Autodesk Inventor part; units mm, degrees
(part 2 of 2)
sketch "Sketch8" plane through (0, 0, 9) normal (0, 0, -1) x (-1, 0, 0)
  circle A0 centre (-8.9909, 76.1845) radius 2.5 projected
  circle A1 centre (-46.3909, 76.1845) radius 2.5 projected
  circle A2 centre (-27.6909, 76.1845) radius 2.5 projected
  arc A3 (-14.3665, 90.3268) -> (-12.2661, 92.4931) centre (-15.59, 93.6145) ccw projected
  arc A4 (-14.955, 86.1395) -> (-14.3665, 90.3268) centre (-14.955, 88.2745) ccw projected
  line L0 (-17.86, 86.1395) -> (-14.955, 86.1395) projected
  line L1 (-17.86, 86.6395) -> (-17.86, 86.1395) projected
  line L2 (-14.955, 86.6395) -> (-17.86, 86.6395) projected
  arc A5 (-14.955, 86.6395) -> (-14.955, 89.9095) centre (-14.955, 88.2745) ccw projected
  line L3 (-16.225, 89.9095) -> (-14.955, 89.9095) projected
  arc A6 (-16.7766, 90.8591) -> (-16.225, 89.9095) centre (-16.225, 90.5445) ccw projected
  arc A7 (-16.7766, 90.8591) -> (-12.6611, 92.9653) centre (-15.59, 93.6145) ccw projected
  arc A8 (-12.6611, 92.9653) -> (-11.1978, 95.4171) centre (-12.6138, 94.5996) ccw projected
  line L4 (-11.8328, 96.5169) -> (-11.1978, 95.4171) projected
  arc A9 (-10.733, 97.1519) -> (-11.8328, 96.5169) centre (-11.2829, 96.8344) ccw projected
  line L5 (-9.2805, 94.6361) -> (-10.733, 97.1519) projected
  line L6 (-9.7135, 94.3861) -> (-9.2805, 94.6361) projected
  line L7 (-11.157, 93.0388) -> (-9.7135, 94.3861) projected
  arc A10 (-12.2661, 92.4931) -> (-11.157, 93.0388) centre (-12.6138, 94.5996) ccw projected
  arc A11 (-19.049, 94.1988) -> (-18.2231, 91.2966) centre (-15.59, 93.6145) ccw projected
  arc A12 (-22.3811, 96.8021) -> (-19.049, 94.1988) centre (-20.5321, 95.7346) ccw projected
  line L8 (-20.9286, 99.3179) -> (-22.3811, 96.8021) projected
  line L9 (-20.4955, 99.0679) -> (-20.9286, 99.3179) projected
  line L10 (-21.948, 96.5521) -> (-20.4955, 99.0679) projected
  arc A13 (-21.948, 96.5521) -> (-19.1161, 94.9171) centre (-20.5321, 95.7346) ccw projected
  line L11 (-18.4811, 96.0169) -> (-19.1161, 94.9171) projected
  arc A14 (-17.3829, 96.0198) -> (-18.4811, 96.0169) centre (-17.9312, 95.6994) ccw projected
  arc A15 (-17.3829, 96.0198) -> (-17.6167, 91.4026) centre (-15.59, 93.6145) ccw projected
  arc A16 (-17.6167, 91.4026) -> (-16.225, 88.9095) centre (-16.225, 90.5445) ccw projected
  line L12 (-14.955, 88.9095) -> (-16.225, 88.9095) projected
  arc A17 (-14.955, 87.6395) -> (-14.955, 88.9095) centre (-14.955, 88.2745) ccw projected
  line L13 (-17.86, 87.6395) -> (-14.955, 87.6395) projected
  line L14 (-17.86, 88.1395) -> (-17.86, 87.6395) projected
  line L15 (-18.3051, 90.0633) -> (-17.86, 88.1395) projected
  arc A18 (-18.2231, 91.2966) -> (-18.3051, 90.0633) centre (-16.225, 90.5445) ccw projected
  arc A19 (-13.3545, 96.3179) -> (-16.2808, 97.0538) centre (-15.59, 93.6145) ccw projected
  arc A20 (-9.4339, 97.9019) -> (-13.3545, 96.3179) centre (-11.2829, 96.8344) ccw projected
  line L16 (-7.9814, 95.3861) -> (-9.4339, 97.9019) projected
  line L17 (-8.4145, 95.1361) -> (-7.9814, 95.3861) projected
  line L18 (-9.867, 97.6519) -> (-8.4145, 95.1361) projected
  arc A21 (-9.867, 97.6519) -> (-12.6989, 96.0169) centre (-11.2829, 96.8344) ccw projected
  line L19 (-12.0639, 94.9171) -> (-12.6989, 96.0169) projected
  arc A22 (-12.6105, 93.9646) -> (-12.0639, 94.9171) centre (-12.6138, 94.5996) ccw projected
  arc A23 (-12.6105, 93.9646) -> (-16.4922, 96.4756) centre (-15.59, 93.6145) ccw projected
  arc A24 (-16.4922, 96.4756) -> (-19.3472, 96.5169) centre (-17.9312, 95.6994) ccw projected
  line L20 (-19.9822, 95.4171) -> (-19.3472, 96.5169) projected
  arc A25 (-21.082, 96.0521) -> (-19.9822, 95.4171) centre (-20.5321, 95.7346) ccw projected
  line L21 (-19.6295, 98.5679) -> (-21.082, 96.0521) projected
  line L22 (-19.1965, 98.3179) -> (-19.6295, 98.5679) projected
  line L23 (-17.3079, 97.7414) -> (-19.1965, 98.3179) projected
  arc A26 (-16.2808, 97.0538) -> (-17.3079, 97.7414) centre (-17.9312, 95.6994) ccw projected
  arc A27 (-33.0665, 90.3268) -> (-30.9661, 92.4931) centre (-34.29, 93.6145) ccw projected
  arc A28 (-33.655, 86.1395) -> (-33.0665, 90.3268) centre (-33.655, 88.2745) ccw projected
  line L24 (-36.56, 86.1395) -> (-33.655, 86.1395) projected
  line L25 (-36.56, 86.6395) -> (-36.56, 86.1395) projected
  line L26 (-33.655, 86.6395) -> (-36.56, 86.6395) projected
  arc A29 (-33.655, 86.6395) -> (-33.655, 89.9095) centre (-33.655, 88.2745) ccw projected
  line L27 (-34.925, 89.9095) -> (-33.655, 89.9095) projected
  arc A30 (-35.4766, 90.8591) -> (-34.925, 89.9095) centre (-34.925, 90.5445) ccw projected
  arc A31 (-35.4766, 90.8591) -> (-31.3611, 92.9653) centre (-34.29, 93.6145) ccw projected
  arc A32 (-31.3611, 92.9653) -> (-29.8978, 95.4171) centre (-31.3138, 94.5996) ccw projected
  line L28 (-30.5328, 96.5169) -> (-29.8978, 95.4171) projected
  arc A33 (-29.433, 97.1519) -> (-30.5328, 96.5169) centre (-29.9829, 96.8344) ccw projected
  line L29 (-27.9805, 94.6361) -> (-29.433, 97.1519) projected
  line L30 (-28.4135, 94.3861) -> (-27.9805, 94.6361) projected
  line L31 (-29.857, 93.0388) -> (-28.4135, 94.3861) projected
  arc A34 (-30.9661, 92.4931) -> (-29.857, 93.0388) centre (-31.3138, 94.5996) ccw projected
  arc A35 (-37.749, 94.1988) -> (-36.9231, 91.2966) centre (-34.29, 93.6145) ccw projected
  arc A36 (-41.0811, 96.8021) -> (-37.749, 94.1988) centre (-39.2321, 95.7346) ccw projected
  line L32 (-39.6286, 99.3179) -> (-41.0811, 96.8021) projected
  line L33 (-39.1955, 99.0679) -> (-39.6286, 99.3179) projected
  line L34 (-40.648, 96.5521) -> (-39.1955, 99.0679) projected
  arc A37 (-40.648, 96.5521) -> (-37.8161, 94.9171) centre (-39.2321, 95.7346) ccw projected
  line L35 (-37.1811, 96.0169) -> (-37.8161, 94.9171) projected
  arc A38 (-36.0829, 96.0198) -> (-37.1811, 96.0169) centre (-36.6312, 95.6994) ccw projected
  arc A39 (-36.0829, 96.0198) -> (-36.3167, 91.4026) centre (-34.29, 93.6145) ccw projected
  arc A40 (-36.3167, 91.4026) -> (-34.925, 88.9095) centre (-34.925, 90.5445) ccw projected
  line L36 (-33.655, 88.9095) -> (-34.925, 88.9095) projected
  arc A41 (-33.655, 87.6395) -> (-33.655, 88.9095) centre (-33.655, 88.2745) ccw projected
  line L37 (-36.56, 87.6395) -> (-33.655, 87.6395) projected
  line L38 (-36.56, 88.1395) -> (-36.56, 87.6395) projected
  line L39 (-37.0051, 90.0633) -> (-36.56, 88.1395) projected
  arc A42 (-36.9231, 91.2966) -> (-37.0051, 90.0633) centre (-34.925, 90.5445) ccw projected
  arc A43 (-32.0545, 96.3179) -> (-34.9808, 97.0538) centre (-34.29, 93.6145) ccw projected
  arc A44 (-28.1339, 97.9019) -> (-32.0545, 96.3179) centre (-29.9829, 96.8344) ccw projected
  line L40 (-26.6814, 95.3861) -> (-28.1339, 97.9019) projected
  line L41 (-27.1145, 95.1361) -> (-26.6814, 95.3861) projected
  line L42 (-28.567, 97.6519) -> (-27.1145, 95.1361) projected
  arc A45 (-28.567, 97.6519) -> (-31.3989, 96.0169) centre (-29.9829, 96.8344) ccw projected
  line L43 (-30.7639, 94.9171) -> (-31.3989, 96.0169) projected
  arc A46 (-31.3105, 93.9646) -> (-30.7639, 94.9171) centre (-31.3138, 94.5996) ccw projected
  arc A47 (-31.3105, 93.9646) -> (-35.1922, 96.4756) centre (-34.29, 93.6145) ccw projected
  arc A48 (-35.1922, 96.4756) -> (-38.0472, 96.5169) centre (-36.6312, 95.6994) ccw projected
  line L44 (-38.6822, 95.4171) -> (-38.0472, 96.5169) projected
  arc A49 (-39.782, 96.0521) -> (-38.6822, 95.4171) centre (-39.2321, 95.7346) ccw projected
  line L45 (-38.3295, 98.5679) -> (-39.782, 96.0521) projected
  line L46 (-37.8965, 98.3179) -> (-38.3295, 98.5679) projected
  line L47 (-36.0079, 97.7414) -> (-37.8965, 98.3179) projected
  arc A50 (-34.9808, 97.0538) -> (-36.0079, 97.7414) centre (-36.6312, 95.6994) ccw projected
  arc A51 (-51.7665, 90.3268) -> (-49.6661, 92.4931) centre (-52.99, 93.6145) ccw projected
  arc A52 (-52.355, 86.1395) -> (-51.7665, 90.3268) centre (-52.355, 88.2745) ccw projected
  line L48 (-55.26, 86.1395) -> (-52.355, 86.1395) projected
  line L49 (-55.26, 86.6395) -> (-55.26, 86.1395) projected
  line L50 (-52.355, 86.6395) -> (-55.26, 86.6395) projected
  arc A53 (-52.355, 86.6395) -> (-52.355, 89.9095) centre (-52.355, 88.2745) ccw projected
  line L51 (-53.625, 89.9095) -> (-52.355, 89.9095) projected
  arc A54 (-54.1766, 90.8591) -> (-53.625, 89.9095) centre (-53.625, 90.5445) ccw projected
  arc A55 (-54.1766, 90.8591) -> (-50.0611, 92.9653) centre (-52.99, 93.6145) ccw projected
  arc A56 (-50.0611, 92.9653) -> (-48.5978, 95.4171) centre (-50.0138, 94.5996) ccw projected
  line L52 (-49.2328, 96.5169) -> (-48.5978, 95.4171) projected
  arc A57 (-48.133, 97.1519) -> (-49.2328, 96.5169) centre (-48.6829, 96.8344) ccw projected
  line L53 (-46.6805, 94.6361) -> (-48.133, 97.1519) projected
  line L54 (-47.1135, 94.3861) -> (-46.6805, 94.6361) projected
  line L55 (-48.557, 93.0388) -> (-47.1135, 94.3861) projected
  arc A58 (-49.6661, 92.4931) -> (-48.557, 93.0388) centre (-50.0138, 94.5996) ccw projected
  arc A59 (-56.449, 94.1988) -> (-55.6231, 91.2966) centre (-52.99, 93.6145) ccw projected
  arc A60 (-59.7811, 96.8021) -> (-56.449, 94.1988) centre (-57.9321, 95.7346) ccw projected
  line L56 (-58.3286, 99.3179) -> (-59.7811, 96.8021) projected
  line L57 (-57.8955, 99.0679) -> (-58.3286, 99.3179) projected
  line L58 (-59.348, 96.5521) -> (-57.8955, 99.0679) projected
  arc A61 (-59.348, 96.5521) -> (-56.5161, 94.9171) centre (-57.9321, 95.7346) ccw projected
  line L59 (-55.8811, 96.0169) -> (-56.5161, 94.9171) projected
  arc A62 (-54.7829, 96.0198) -> (-55.8811, 96.0169) centre (-55.3312, 95.6994) ccw projected
  arc A63 (-54.7829, 96.0198) -> (-55.0167, 91.4026) centre (-52.99, 93.6145) ccw projected
  arc A64 (-55.0167, 91.4026) -> (-53.625, 88.9095) centre (-53.625, 90.5445) ccw projected
  line L60 (-52.355, 88.9095) -> (-53.625, 88.9095) projected
  arc A65 (-52.355, 87.6395) -> (-52.355, 88.9095) centre (-52.355, 88.2745) ccw projected
  line L61 (-55.26, 87.6395) -> (-52.355, 87.6395) projected
  line L62 (-55.26, 88.1395) -> (-55.26, 87.6395) projected
  line L63 (-55.7051, 90.0633) -> (-55.26, 88.1395) projected
  arc A66 (-55.6231, 91.2966) -> (-55.7051, 90.0633) centre (-53.625, 90.5445) ccw projected
  arc A67 (-50.7545, 96.3179) -> (-53.6808, 97.0538) centre (-52.99, 93.6145) ccw projected
  arc A68 (-46.8339, 97.9019) -> (-50.7545, 96.3179) centre (-48.6829, 96.8344) ccw projected
  line L64 (-45.3814, 95.3861) -> (-46.8339, 97.9019) projected
  line L65 (-45.8145, 95.1361) -> (-45.3814, 95.3861) projected
  line L66 (-47.267, 97.6519) -> (-45.8145, 95.1361) projected
  arc A69 (-47.267, 97.6519) -> (-50.0989, 96.0169) centre (-48.6829, 96.8344) ccw projected
  line L67 (-49.4639, 94.9171) -> (-50.0989, 96.0169) projected
  arc A70 (-50.0105, 93.9646) -> (-49.4639, 94.9171) centre (-50.0138, 94.5996) ccw projected
  arc A71 (-50.0105, 93.9646) -> (-53.8922, 96.4756) centre (-52.99, 93.6145) ccw projected
  arc A72 (-53.8922, 96.4756) -> (-56.7472, 96.5169) centre (-55.3312, 95.6994) ccw projected
  line L68 (-57.3822, 95.4171) -> (-56.7472, 96.5169) projected
  arc A73 (-58.482, 96.0521) -> (-57.3822, 95.4171) centre (-57.9321, 95.7346) ccw projected
  line L69 (-57.0295, 98.5679) -> (-58.482, 96.0521) projected
  line L70 (-56.5965, 98.3179) -> (-57.0295, 98.5679) projected
  line L71 (-54.7079, 97.7414) -> (-56.5965, 98.3179) projected
  arc A74 (-53.6808, 97.0538) -> (-54.7079, 97.7414) centre (-55.3312, 95.6994) ccw projected
  arc A75 (-14.3665, 76.7068) -> (-12.2661, 78.8731) centre (-15.59, 79.9945) ccw projected
  arc A76 (-14.955, 72.5195) -> (-14.3665, 76.7068) centre (-14.955, 74.6545) ccw projected
  line L72 (-17.86, 72.5195) -> (-14.955, 72.5195) projected
  line L73 (-17.86, 73.0195) -> (-17.86, 72.5195) projected
  line L74 (-14.955, 73.0195) -> (-17.86, 73.0195) projected
  arc A77 (-14.955, 73.0195) -> (-14.955, 76.2895) centre (-14.955, 74.6545) ccw projected
  line L75 (-16.225, 76.2895) -> (-14.955, 76.2895) projected
  arc A78 (-16.7766, 77.2391) -> (-16.225, 76.2895) centre (-16.225, 76.9245) ccw projected
  arc A79 (-16.7766, 77.2391) -> (-12.6611, 79.3453) centre (-15.59, 79.9945) ccw projected
  arc A80 (-12.6611, 79.3453) -> (-11.1978, 81.7971) centre (-12.6138, 80.9796) ccw projected
  line L76 (-11.8328, 82.8969) -> (-11.1978, 81.7971) projected
  arc A81 (-10.733, 83.5319) -> (-11.8328, 82.8969) centre (-11.2829, 83.2144) ccw projected
  line L77 (-9.2805, 81.0161) -> (-10.733, 83.5319) projected
  line L78 (-9.7135, 80.7661) -> (-9.2805, 81.0161) projected
  line L79 (-11.157, 79.4188) -> (-9.7135, 80.7661) projected
  arc A82 (-12.2661, 78.8731) -> (-11.157, 79.4188) centre (-12.6138, 80.9796) ccw projected
  arc A83 (-19.049, 80.5788) -> (-18.2231, 77.6766) centre (-15.59, 79.9945) ccw projected
  arc A84 (-22.3811, 83.1821) -> (-19.049, 80.5788) centre (-20.5321, 82.1146) ccw projected
  line L80 (-20.9286, 85.6979) -> (-22.3811, 83.1821) projected
  line L81 (-20.4955, 85.4479) -> (-20.9286, 85.6979) projected
  line L82 (-21.948, 82.9321) -> (-20.4955, 85.4479) projected
  arc A85 (-21.948, 82.9321) -> (-19.1161, 81.2971) centre (-20.5321, 82.1146) ccw projected
  line L83 (-18.4811, 82.3969) -> (-19.1161, 81.2971) projected
  arc A86 (-17.3829, 82.3998) -> (-18.4811, 82.3969) centre (-17.9312, 82.0794) ccw projected
  arc A87 (-17.3829, 82.3998) -> (-17.6167, 77.7826) centre (-15.59, 79.9945) ccw projected
  arc A88 (-17.6167, 77.7826) -> (-16.225, 75.2895) centre (-16.225, 76.9245) ccw projected
  line L84 (-14.955, 75.2895) -> (-16.225, 75.2895) projected
  arc A89 (-14.955, 74.0195) -> (-14.955, 75.2895) centre (-14.955, 74.6545) ccw projected
  line L85 (-17.86, 74.0195) -> (-14.955, 74.0195) projected
  line L86 (-17.86, 74.5195) -> (-17.86, 74.0195) projected
  line L87 (-18.3051, 76.4433) -> (-17.86, 74.5195) projected
  arc A90 (-18.2231, 77.6766) -> (-18.3051, 76.4433) centre (-16.225, 76.9245) ccw projected
  arc A91 (-13.3545, 82.6979) -> (-16.2808, 83.4338) centre (-15.59, 79.9945) ccw projected
  arc A92 (-9.4339, 84.2819) -> (-13.3545, 82.6979) centre (-11.2829, 83.2144) ccw projected
  line L88 (-7.9814, 81.7661) -> (-9.4339, 84.2819) projected
  line L89 (-8.4145, 81.5161) -> (-7.9814, 81.7661) projected
  line L90 (-9.867, 84.0319) -> (-8.4145, 81.5161) projected
  arc A93 (-9.867, 84.0319) -> (-12.6989, 82.3969) centre (-11.2829, 83.2144) ccw projected
  line L91 (-12.0639, 81.2971) -> (-12.6989, 82.3969) projected
  arc A94 (-12.6105, 80.3446) -> (-12.0639, 81.2971) centre (-12.6138, 80.9796) ccw projected
  arc A95 (-12.6105, 80.3446) -> (-16.4922, 82.8556) centre (-15.59, 79.9945) ccw projected
  arc A96 (-16.4922, 82.8556) -> (-19.3472, 82.8969) centre (-17.9312, 82.0794) ccw projected
  line L92 (-19.9822, 81.7971) -> (-19.3472, 82.8969) projected
  arc A97 (-21.082, 82.4321) -> (-19.9822, 81.7971) centre (-20.5321, 82.1146) ccw projected
  line L93 (-19.6295, 84.9479) -> (-21.082, 82.4321) projected
  line L94 (-19.1965, 84.6979) -> (-19.6295, 84.9479) projected
  line L95 (-17.3079, 84.1214) -> (-19.1965, 84.6979) projected
  arc A98 (-16.2808, 83.4338) -> (-17.3079, 84.1214) centre (-17.9312, 82.0794) ccw projected
  arc A99 (-33.0665, 76.7068) -> (-30.9661, 78.8731) centre (-34.29, 79.9945) ccw projected
  arc A100 (-33.655, 72.5195) -> (-33.0665, 76.7068) centre (-33.655, 74.6545) ccw projected
  line L96 (-36.56, 72.5195) -> (-33.655, 72.5195) projected
  line L97 (-36.56, 73.0195) -> (-36.56, 72.5195) projected
  line L98 (-33.655, 73.0195) -> (-36.56, 73.0195) projected
  arc A101 (-33.655, 73.0195) -> (-33.655, 76.2895) centre (-33.655, 74.6545) ccw projected
  line L99 (-34.925, 76.2895) -> (-33.655, 76.2895) projected
  arc A102 (-35.4766, 77.2391) -> (-34.925, 76.2895) centre (-34.925, 76.9245) ccw projected
  arc A103 (-35.4766, 77.2391) -> (-31.3611, 79.3453) centre (-34.29, 79.9945) ccw projected
  arc A104 (-31.3611, 79.3453) -> (-29.8978, 81.7971) centre (-31.3138, 80.9796) ccw projected
  line L100 (-30.5328, 82.8969) -> (-29.8978, 81.7971) projected
  arc A105 (-29.433, 83.5319) -> (-30.5328, 82.8969) centre (-29.9829, 83.2144) ccw projected
  line L101 (-27.9805, 81.0161) -> (-29.433, 83.5319) projected
  line L102 (-28.4135, 80.7661) -> (-27.9805, 81.0161) projected
  line L103 (-29.857, 79.4188) -> (-28.4135, 80.7661) projected
  arc A106 (-30.9661, 78.8731) -> (-29.857, 79.4188) centre (-31.3138, 80.9796) ccw projected
  arc A107 (-37.749, 80.5788) -> (-36.9231, 77.6766) centre (-34.29, 79.9945) ccw projected
  arc A108 (-41.0811, 83.1821) -> (-37.749, 80.5788) centre (-39.2321, 82.1146) ccw projected
  line L104 (-39.6286, 85.6979) -> (-41.0811, 83.1821) projected
  line L105 (-39.1955, 85.4479) -> (-39.6286, 85.6979) projected
  line L106 (-40.648, 82.9321) -> (-39.1955, 85.4479) projected
  arc A109 (-40.648, 82.9321) -> (-37.8161, 81.2971) centre (-39.2321, 82.1146) ccw projected
  line L107 (-37.1811, 82.3969) -> (-37.8161, 81.2971) projected
  arc A110 (-36.0829, 82.3998) -> (-37.1811, 82.3969) centre (-36.6312, 82.0794) ccw projected
  arc A111 (-36.0829, 82.3998) -> (-36.3167, 77.7826) centre (-34.29, 79.9945) ccw projected
  arc A112 (-36.3167, 77.7826) -> (-34.925, 75.2895) centre (-34.925, 76.9245) ccw projected
  line L108 (-33.655, 75.2895) -> (-34.925, 75.2895) projected
  arc A113 (-33.655, 74.0195) -> (-33.655, 75.2895) centre (-33.655, 74.6545) ccw projected
  line L109 (-36.56, 74.0195) -> (-33.655, 74.0195) projected
  line L110 (-36.56, 74.5195) -> (-36.56, 74.0195) projected
  line L111 (-37.0051, 76.4433) -> (-36.56, 74.5195) projected
  arc A114 (-36.9231, 77.6766) -> (-37.0051, 76.4433) centre (-34.925, 76.9245) ccw projected
  arc A115 (-32.0545, 82.6979) -> (-34.9808, 83.4338) centre (-34.29, 79.9945) ccw projected
  arc A116 (-28.1339, 84.2819) -> (-32.0545, 82.6979) centre (-29.9829, 83.2144) ccw projected
  line L112 (-26.6814, 81.7661) -> (-28.1339, 84.2819) projected
  line L113 (-27.1145, 81.5161) -> (-26.6814, 81.7661) projected
  line L114 (-28.567, 84.0319) -> (-27.1145, 81.5161) projected
  arc A117 (-28.567, 84.0319) -> (-31.3989, 82.3969) centre (-29.9829, 83.2144) ccw projected
  line L115 (-30.7639, 81.2971) -> (-31.3989, 82.3969) projected
  arc A118 (-31.3105, 80.3446) -> (-30.7639, 81.2971) centre (-31.3138, 80.9796) ccw projected
  arc A119 (-31.3105, 80.3446) -> (-35.1922, 82.8556) centre (-34.29, 79.9945) ccw projected
  arc A120 (-35.1922, 82.8556) -> (-38.0472, 82.8969) centre (-36.6312, 82.0794) ccw projected
  line L116 (-38.6822, 81.7971) -> (-38.0472, 82.8969) projected
  arc A121 (-39.782, 82.4321) -> (-38.6822, 81.7971) centre (-39.2321, 82.1146) ccw projected
  line L117 (-38.3295, 84.9479) -> (-39.782, 82.4321) projected
  line L118 (-37.8965, 84.6979) -> (-38.3295, 84.9479) projected
  line L119 (-36.0079, 84.1214) -> (-37.8965, 84.6979) projected
  arc A122 (-34.9808, 83.4338) -> (-36.0079, 84.1214) centre (-36.6312, 82.0794) ccw projected
  arc A123 (-56.449, 80.5788) -> (-55.6231, 77.6766) centre (-52.99, 79.9945) ccw projected
  arc A124 (-59.7811, 83.1821) -> (-56.449, 80.5788) centre (-57.9321, 82.1146) ccw projected
  line L120 (-58.3286, 85.6979) -> (-59.7811, 83.1821) projected
  line L121 (-57.8955, 85.4479) -> (-58.3286, 85.6979) projected
  line L122 (-59.348, 82.9321) -> (-57.8955, 85.4479) projected
  arc A125 (-59.348, 82.9321) -> (-56.5161, 81.2971) centre (-57.9321, 82.1146) ccw projected
  line L123 (-55.8811, 82.3969) -> (-56.5161, 81.2971) projected
  arc A126 (-54.7829, 82.3998) -> (-55.8811, 82.3969) centre (-55.3312, 82.0794) ccw projected
  arc A127 (-54.7829, 82.3998) -> (-55.0167, 77.7826) centre (-52.99, 79.9945) ccw projected
  arc A128 (-55.0167, 77.7826) -> (-53.625, 75.2895) centre (-53.625, 76.9245) ccw projected
  line L124 (-52.355, 75.2895) -> (-53.625, 75.2895) projected
  arc A129 (-52.355, 74.0195) -> (-52.355, 75.2895) centre (-52.355, 74.6545) ccw projected
  line L125 (-55.26, 74.0195) -> (-52.355, 74.0195) projected
  line L126 (-55.26, 74.5195) -> (-55.26, 74.0195) projected
  line L127 (-55.7051, 76.4433) -> (-55.26, 74.5195) projected
  arc A130 (-55.6231, 77.6766) -> (-55.7051, 76.4433) centre (-53.625, 76.9245) ccw projected
  arc A131 (-50.0105, 80.3446) -> (-53.8922, 82.8556) centre (-52.99, 79.9945) ccw projected
  arc A132 (-53.8922, 82.8556) -> (-56.7472, 82.8969) centre (-55.3312, 82.0794) ccw projected
  line L128 (-57.3822, 81.7971) -> (-56.7472, 82.8969) projected
  arc A133 (-58.482, 82.4321) -> (-57.3822, 81.7971) centre (-57.9321, 82.1146) ccw projected
  line L129 (-57.0295, 84.9479) -> (-58.482, 82.4321) projected
  line L130 (-56.5965, 84.6979) -> (-57.0295, 84.9479) projected
  line L131 (-54.7079, 84.1214) -> (-56.5965, 84.6979) projected
  arc A134 (-53.6808, 83.4338) -> (-54.7079, 84.1214) centre (-55.3312, 82.0794) ccw projected
  arc A135 (-50.7545, 82.6979) -> (-53.6808, 83.4338) centre (-52.99, 79.9945) ccw projected
  arc A136 (-46.8339, 84.2819) -> (-50.7545, 82.6979) centre (-48.6829, 83.2144) ccw projected
  line L132 (-45.3814, 81.7661) -> (-46.8339, 84.2819) projected
  line L133 (-45.8145, 81.5161) -> (-45.3814, 81.7661) projected
  line L134 (-47.267, 84.0319) -> (-45.8145, 81.5161) projected
  arc A137 (-47.267, 84.0319) -> (-50.0989, 82.3969) centre (-48.6829, 83.2144) ccw projected
  line L135 (-49.4639, 81.2971) -> (-50.0989, 82.3969) projected
  arc A138 (-50.0105, 80.3446) -> (-49.4639, 81.2971) centre (-50.0138, 80.9796) ccw projected
  arc A139 (-50.0611, 79.3453) -> (-48.5978, 81.7971) centre (-50.0138, 80.9796) ccw projected
  line L136 (-49.2328, 82.8969) -> (-48.5978, 81.7971) projected
  arc A140 (-48.133, 83.5319) -> (-49.2328, 82.8969) centre (-48.6829, 83.2144) ccw projected
  line L137 (-46.6805, 81.0161) -> (-48.133, 83.5319) projected
  line L138 (-47.1135, 80.7661) -> (-46.6805, 81.0161) projected
  line L139 (-48.557, 79.4188) -> (-47.1135, 80.7661) projected
  arc A141 (-49.6661, 78.8731) -> (-48.557, 79.4188) centre (-50.0138, 80.9796) ccw projected
  arc A142 (-51.7665, 76.7068) -> (-49.6661, 78.8731) centre (-52.99, 79.9945) ccw projected
  arc A143 (-52.355, 72.5195) -> (-51.7665, 76.7068) centre (-52.355, 74.6545) ccw projected
  line L140 (-55.26, 72.5195) -> (-52.355, 72.5195) projected
  line L141 (-55.26, 73.0195) -> (-55.26, 72.5195) projected
  line L142 (-52.355, 73.0195) -> (-55.26, 73.0195) projected
  arc A144 (-52.355, 73.0195) -> (-52.355, 76.2895) centre (-52.355, 74.6545) ccw projected
  line L143 (-53.625, 76.2895) -> (-52.355, 76.2895) projected
  arc A145 (-54.1766, 77.2391) -> (-53.625, 76.2895) centre (-53.625, 76.9245) ccw projected
  arc A146 (-54.1766, 77.2391) -> (-50.0611, 79.3453) centre (-52.99, 79.9945) ccw projected
  line L144 (-2, 65.8874) -> (-66.58, 65.8874) projected
  line L145 (-2, 105.95) -> (-2, 65.8874) projected
  line L146 (-66.58, 105.95) -> (-2, 105.95) projected
  line L147 (-66.58, 65.8874) -> (-66.58, 105.95) projected
  line L148 (-9.7135, 80.7661) -> (-9.2805, 81.0161) projected
  line L149 (-9.2805, 81.0161) -> (-8.4145, 81.5161)
  line L150 (-17.86, 73.0195) -> (-17.86, 72.5195) projected
  line L151 (-17.86, 74.0195) -> (-17.86, 73.0195)
  line L152 (-20.4955, 85.4479) -> (-20.9286, 85.6979) projected
  line L153 (-20.4955, 85.4479) -> (-19.6295, 84.9479)
  line L154 (-8.4145, 95.1361) -> (-7.9814, 95.3861) projected
  line L155 (-8.4145, 95.1361) -> (-9.2805, 94.6361)
  line L156 (-17.86, 86.6395) -> (-17.86, 86.1395) projected
  line L157 (-17.86, 87.6395) -> (-17.86, 86.6395)
  line L158 (-20.4955, 99.0679) -> (-19.6295, 98.5679)
  line L159 (-27.1145, 95.1361) -> (-26.6814, 95.3861) projected
  line L160 (-27.1145, 95.1361) -> (-27.9805, 94.6361)
  line L161 (-27.1145, 81.5161) -> (-27.9805, 81.0161)
  line L162 (-36.56, 73.0195) -> (-36.56, 72.5195) projected
  line L163 (-36.56, 74.0195) -> (-36.56, 73.0195)
  line L164 (-40.648, 82.9321) -> (-39.1955, 85.4479) projected
  line L165 (-38.3295, 84.9479) -> (-39.1955, 85.4479)
  line L166 (-33.655, 86.6395) -> (-36.56, 86.6395) projected
  line L167 (-36.56, 86.6395) -> (-36.56, 87.6395)
  line L168 (-40.648, 96.5521) -> (-39.1955, 99.0679) projected
  line L169 (-39.1955, 99.0679) -> (-38.3295, 98.5679)
  line L170 (-46.6805, 81.0161) -> (-45.8145, 81.5161)
  line L171 (-55.26, 73.0195) -> (-55.26, 72.5195) projected
  line L172 (-55.26, 73.0195) -> (-55.26, 74.0195)
  line L173 (-57.8955, 85.4479) -> (-57.0295, 84.9479)
  line L174 (-55.26, 87.6395) -> (-55.26, 86.6395)
  line L175 (-45.8145, 95.1361) -> (-45.3814, 95.3861) projected
  line L176 (-45.8145, 95.1361) -> (-46.6805, 94.6361)
  line L177 (-59.348, 96.5521) -> (-57.8955, 99.0679) projected
  line L178 (-57.0295, 98.5679) -> (-58.482, 96.0521) projected
  line L179 (-57.8955, 99.0679) -> (-57.0295, 98.5679)
  line L180 (-37.29, 82.9945) -> (-31.29, 82.9945)
  line L181 (-31.29, 82.9945) -> (-31.29, 76.9945)
  line L182 (-31.29, 76.9945) -> (-37.29, 76.9945)
  line L183 (-37.29, 76.9945) -> (-37.29, 82.9945)
  line L184 (-37.29, 82.9945) -> (-31.29, 76.9945) construction
  line L185 (-31.29, 82.9945) -> (-37.29, 76.9945) construction
  line L186 (-37.29, 96.6145) -> (-31.29, 96.6145)
  line L187 (-31.29, 96.6145) -> (-31.29, 90.6145)
  line L188 (-31.29, 90.6145) -> (-37.29, 90.6145)
  line L189 (-37.29, 90.6145) -> (-37.29, 96.6145)
  line L190 (-37.29, 96.6145) -> (-31.29, 90.6145) construction
  line L191 (-31.29, 96.6145) -> (-37.29, 90.6145) construction
  line L192 (-12.59, 96.6145) -> (-18.59, 96.6145)
  line L193 (-18.59, 96.6145) -> (-18.59, 90.6145)
  line L194 (-18.59, 90.6145) -> (-12.59, 90.6145)
  line L195 (-12.59, 90.6145) -> (-12.59, 96.6145)
  line L196 (-12.59, 96.6145) -> (-18.59, 90.6145) construction
  line L197 (-18.59, 96.6145) -> (-12.59, 90.6145) construction
  line L198 (-12.59, 82.9945) -> (-18.59, 82.9945)
  line L199 (-18.59, 82.9945) -> (-18.59, 76.9945)
  line L200 (-18.59, 76.9945) -> (-12.59, 76.9945)
  line L201 (-12.59, 76.9945) -> (-12.59, 82.9945)
  line L202 (-12.59, 82.9945) -> (-18.59, 76.9945) construction
  line L203 (-18.59, 82.9945) -> (-12.59, 76.9945) construction
  line L204 (-49.99, 82.9945) -> (-55.99, 82.9945)
  line L205 (-55.99, 82.9945) -> (-55.99, 76.9945)
  line L206 (-55.99, 76.9945) -> (-49.99, 76.9945)
  line L207 (-49.99, 76.9945) -> (-49.99, 82.9945)
  line L208 (-49.99, 82.9945) -> (-55.99, 76.9945) construction
  line L209 (-55.99, 82.9945) -> (-49.99, 76.9945) construction
  line L210 (-49.99, 96.6145) -> (-55.99, 96.6145)
  line L211 (-55.99, 96.6145) -> (-55.99, 90.6145)
  line L212 (-55.99, 90.6145) -> (-49.99, 90.6145)
  line L213 (-49.99, 90.6145) -> (-49.99, 96.6145)
  line L214 (-49.99, 96.6145) -> (-55.99, 90.6145) construction
  line L215 (-55.99, 96.6145) -> (-49.99, 90.6145) construction
  point P0 (0, 0)
  point P1 (-37.0589, 90.6145)
  point P2 (-37.29, 91.7962)
  point P3 (-32.4717, 96.6145)
  point P4 (-32.1066, 96.6145)
  point P5 (-31.29, 91.7962)
  point P6 (-32.4717, 90.6145)
  point P7 (-37.0589, 76.9945)
  point P8 (-37.29, 78.1762)
  point P9 (-32.4717, 82.9945)
  point P10 (-32.1066, 82.9945)
  point P11 (-31.29, 78.1762)
  point P12 (-32.4717, 76.9945)
  point P13 (-51.1717, 82.9945)
  point P14 (-50.8066, 82.9945)
  point P15 (-49.99, 78.1762)
  point P16 (-51.1717, 76.9945)
  point P17 (-55.7589, 76.9945)
  point P18 (-55.99, 78.1762)
  point P19 (-18.3589, 76.9945)
  point P20 (-18.59, 78.1762)
  point P21 (-13.7717, 82.9945)
  point P22 (-13.4066, 82.9945)
  point P23 (-12.59, 78.1762)
  point P24 (-13.7717, 76.9945)
  point P25 (-55.7589, 90.6145)
  point P26 (-55.99, 91.7962)
  point P27 (-51.1717, 96.6145)
  point P28 (-50.8066, 96.6145)
  point P29 (-49.99, 91.7962)
  point P30 (-51.1717, 90.6145)
  point P31 (-18.3589, 90.6145)
  point P32 (-18.59, 91.7962)
  point P33 (-13.7717, 96.6145)
  point P34 (-13.4066, 96.6145)
  point P35 (-12.59, 91.7962)
  point P36 (-13.7717, 90.6145)
  dimension "d78" = 6
  dimension "d79" = 6
  dimension "d80" = 6
  dimension "d81" = 6
  dimension "d82" = 6
  dimension "d83" = 6
  dimension "d84" = 6
  dimension "d85" = 6
  dimension "d86" = 6
  dimension "d87" = 6
  dimension "d88" = 6
  dimension "d89" = 6
  constraints: 108 end point, 12 midpoint, 12 parallel, 8 perpendicular, 6 horizontal, 4 vertical, 3 collinear, 1 point on line
  measures "d78" distance of L181.end L182.end
  measures "d79" distance of L180.end L181.end
  measures "d80" distance of L187.end L188.end
  measures "d81" distance of L186.end L187.end
  measures "d82" distance of L194.end L193.end
  measures "d83" distance of L193.end L192.end
  measures "d84" distance of L200.end L199.end
  measures "d85" distance of L199.end L198.end
  measures "d86" distance of L206.end L205.end
  measures "d87" distance of L205.end L204.end
  measures "d88" distance of L212.end L211.end
  measures "d89" distance of L211.end L210.end
extrude "Extrusion10" add sketch "Sketch8" along normal blind 3.5
fillet "Fillet1" radius 5 8 edges at (68.58, 107.95, 5) (0, 107.95, 5) (0, 0, 5) (68.58, 0, 5) (66.58, 105.95, 2.75) (2, 105.95, 2.75) (2, 65.8874, 2.75) (66.58, 65.8874, 2.75)
chamfer "Chamfer1" distance 2 angle 45 8 edges at (34.29, 0, 10) (67.1155, 1.4645, 10) (68.58, 53.975, 10) (67.1155, 106.4855, 10) (34.29, 107.95, 10) (1.4645, 106.4855, 10) (0, 53.975, 10) (1.4645, 1.4645, 10)
sketch "Sketch9" plane through (34.29, 35.56, 4) normal (0, 0, 1) x (1, 0, 0)
  line L0 (0, 25.4139) -> (22.0091, -12.707) construction
  line L1 (22.0091, -12.707) -> (-22.0091, -12.707) construction
  line L2 (-22.0091, -12.707) -> (0, 25.4139) construction
  circle A0 centre (0, 25.4139) radius 2
  circle A1 centre (22.0091, -12.707) radius 2
  circle A2 centre (-22.0091, -12.707) radius 2
  circle A3 centre (0, 0) radius 21.3106 projected
  point P0 (-34.29, -35.56)
  dimension "d94" = 44.0182
  dimension "d95" = 4
  constraints: 6 end point, 4 coincident, 3 centre point, 2 equal radius, 1 horizontal, 7 other
  measures "d94" distance of L0.start L0.end
  measures "d95" diameter of A2
extrude "Extrusion11" cut sketch "Sketch9" against normal through all contours A0 | A1 | A2
equation "\"d17\" = d16"
body "Solid1"
